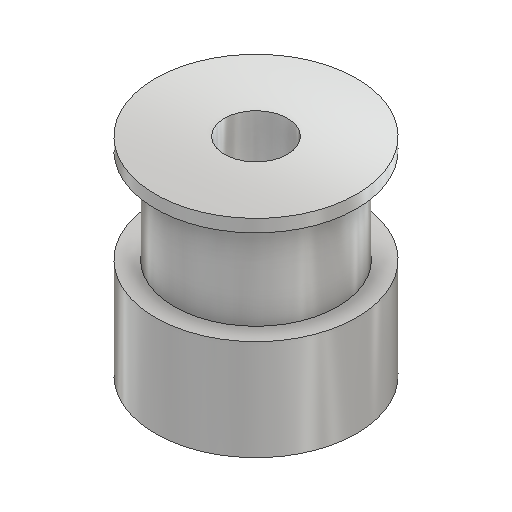
# Autodesk Inventor part: COTS_GENERIC_MXL_Pulley_X_Axis
Saved by Autodesk Inventor 2026.1 (Build 301233000, 233)
## iProperties
Created: 2017-05-29
Part Number: COTS_GENERIC_MXL_Pulley_X_Axis
Material: Ogólny
Document SubType Name: Modeling
Designer: Andrzej
Density: 1 g/cm^3
Appearance: Aluminium - polerowane
Mass: 2.48107 g
Surface Area: 15.1739 cm^2
Volume: 2.48107 cm^3
Author: Andrzej
Autodesk Inventor part; units mm, degrees
ref_plane "YZ Plane" through (0, 0, 0) normal (1, 0, 0) x (0, 1, 0)
ref_plane "XZ Plane" through (0, 0, 0) normal (0, 1, 0) x (-1, 0, 0)
ref_plane "XY Plane" through (0, 0, 0) normal (0, 0, 1) x (1, 0, 0)
sketch "Szkic1" plane through (0, 0, 0) normal (0, 0, 1) x (1, 0, 0)
  circle A0 centre (0, 0) radius 2.5
  circle A1 centre (0, 0) radius 8
  dimension "d0" = 5
  dimension "d1" = 16
  constraints: 2 centre point, 2 coincident
  measures "d0" diameter of A0
  measures "d1" diameter of A1
extrude "Wyciągnięcie proste1" add sketch "Szkic1" along normal blind 8
sketch "Szkic2" plane through (0, 0, 8) normal (0, 0, 1) x (1, 0, 0)
  circle A0 centre (0, 0) radius 2.5 projected
  circle A1 centre (0, 0) radius 8 projected
  circle A2 centre (0, 0) radius 6.5
  dimension "d4" = 13
  constraints: 1 centre point, 1 coincident
  measures "d4" diameter of A2
extrude "Wyciągnięcie proste2" add sketch "Szkic2" along normal blind 7.5 contours A2
sketch "Szkic3" plane through (0, 0, 15.5) normal (0, 0, 1) x (1, 0, 0)
  circle A0 centre (0, 0) radius 6.5 projected
  circle A1 centre (0, 0) radius 8 projected
  circle A2 centre (0, 0) radius 2.5 projected
  circle A3 centre (0, 0) radius 6.5 projected
extrude "Wyciągnięcie proste3" add sketch "Szkic3" along normal blind 1 contours A0 | A1
